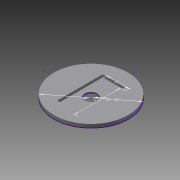
# Autodesk Inventor part: ServoHornBottom
Saved by Autodesk Inventor 2016 (Build 200138000, 138)
## iProperties
Created: 2015-03-17
Part Number: ServoHornBottom
Material: Generic
Document SubType Name: Modeling
Designer: Erin
Density: 1 g/cm^3
Appearance: Default
Author: Erin
Autodesk Inventor part; units mm, degrees
ref_plane "YZ Plane" through (0, 0, 0) normal (1, 0, 0) x (0, 1, 0)
ref_plane "XZ Plane" through (0, 0, 0) normal (0, 1, 0) x (-1, 0, 0)
ref_plane "XY Plane" through (0, 0, 0) normal (0, 0, 1) x (1, 0, 0)
sketch "Sketch1" plane through (0, 0, 0) normal (0, 0, 1) x (1, 0, 0)
  circle A0 centre (0, 0) radius 30
  circle A1 centre (0, 0) radius 5
  line L0 (-9, 18.5) -> (9, 18.5)
  line L1 (9, 18.5) -> (9, -18.5)
  line L2 (9, -18.5) -> (-9, -18.5)
  line L3 (-9, -18.5) -> (-9, 18.5)
  line L4 (0, 0) -> (0, 37.3828) construction
  line L5 (0, 0) -> (-39.0127, 0) construction
  point P0 (0, 18.5)
  point P1 (-9, 0)
  dimension "d0" = 60
  dimension "d1" = 10
  dimension "d2" = 37
  dimension "d3" = 18
  constraints: 12 end point, 3 parallel, 2 centre point, 2 coincident, 2 midpoint, 2 perpendicular, 1 horizontal, 1 horizontal alignment, 1 vertical alignment
  measures "d0" diameter of A0
  measures "d1" diameter of A1
  measures "d2" distance of L0.end L1.end
  measures "d3" distance of L0.start L0.end
extrude "Extrusion1" add sketch "Sketch1" along normal blind 0.6 contours A0 | L0 L1 L2 L3
extrude "Extrusion2" add sketch "Sketch1" along normal blind 2.8 contours A0
body "Solid1"
